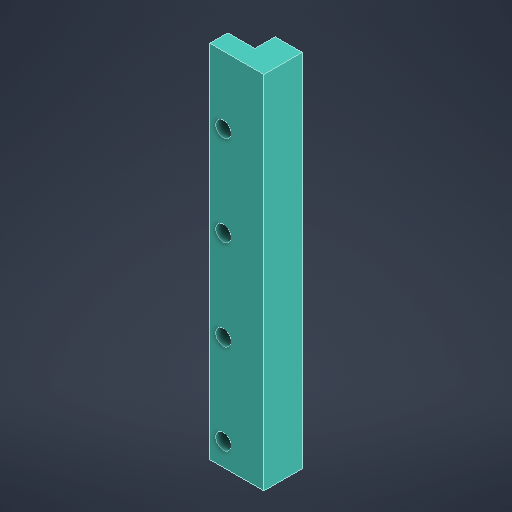
# Autodesk Inventor part: Left_Rod_Support
Saved by Autodesk Inventor 2027.1 (Build 311270010, 270A)
## iProperties
Created: 2026-09-22
Part Number: Left_Rod_Support
Material: Generic
Document SubType Name: Modeling
Designer: 박정현
Density: 1 g/cm^3
Appearance: Left separate support; four original rod clearance holes and four blind M3 x 0.5 - 6H deck threads, 6.5 mm depth.
Author: 박정현
Comments: Left separate support; four original rod clearance holes and four blind M3 x 0.5 - 6H deck threads, 6.5 mm depth.
Autodesk Inventor part; units mm, degrees
ref_plane "Left_Connecting_Web_StartPlane" through (0, 0, 4) normal (0, 0, 1) x (1, 0, 0)
sketch "Left_Connecting_Web_Profile" plane through (0, 0, 4) normal (0, 0, 1) x (1, 0, 0)
  line L0 (6, 0) -> (12, 0)
  line L1 (12, 0) -> (12, 80)
  line L2 (12, 80) -> (6, 80)
  line L3 (6, 80) -> (6, 0)
  point P0 (0, 0)
  dimension "d1" = 6
  dimension "d2" = 6
  dimension "d3" = 80
  constraints: 8 end point, 2 parallel, 1 horizontal, 1 horizontal alignment, 1 perpendicular
  measures "d1" distance of point (0, 0) L0.start
  measures "d2" distance of L1.end L2.end
  measures "d3" distance of L2.end L0.start
extrude "Left_Connecting_Web" add sketch "Left_Connecting_Web_Profile" along normal blind 8.5
ref_plane "Left_Rod_Contact_Flange_StartPlane" through (0, 0, 8.5) normal (0, 0, 1) x (1, 0, 0)
sketch "Left_Rod_Contact_Flange_Profile" plane through (0, 0, 8.5) normal (0, 0, 1) x (1, 0, 0)
  line L0 (0, 0) -> (12, 0)
  line L1 (12, 0) -> (12, 80)
  line L2 (12, 80) -> (0, 80)
  line L3 (0, 80) -> (0, 0)
  dimension "d7" = 12
  dimension "d8" = 80
  constraints: 8 end point, 2 parallel, 1 coincident, 1 horizontal, 1 perpendicular
  measures "d7" distance of L1.end L2.end
  measures "d8" distance of L2.end L0.start
extrude "Left_Rod_Contact_Flange" add sketch "Left_Rod_Contact_Flange_Profile" along normal blind 4
sketch "Original_Rod_Clearance_4x_Locations" plane through (0, 0, 0) normal (0, 0, 1) x (1, 0, 0)
  circle A0 centre (3, 5) radius 1.7
  circle A1 centre (3, 25) radius 1.7
  circle A2 centre (3, 45) radius 1.7
  circle A3 centre (3, 65) radius 1.7
  point P0 (0, 0)
  dimension "d11" = 3
  dimension "d12" = 5
  dimension "d13" = 3.4
  dimension "d14" = 3
  dimension "d15" = 25
  dimension "d16" = 3.4
  dimension "d17" = 3
  dimension "d18" = 45
  dimension "d19" = 3.4
  dimension "d20" = 3
  dimension "d21" = 65
  dimension "d22" = 3.4
  constraints: 4 centre point
  measures "d11" horizontal distance of point (0, 0) A0.centre
  measures "d12" vertical distance of point (0, 0) A0.centre
  measures "d13" diameter of A0
  measures "d14" horizontal distance of point (0, 0) A1.centre
  measures "d15" vertical distance of point (0, 0) A1.centre
  measures "d16" diameter of A1
  measures "d17" horizontal distance of point (0, 0) A2.centre
  measures "d18" vertical distance of point (0, 0) A2.centre
  measures "d19" diameter of A2
  measures "d20" horizontal distance of point (0, 0) A3.centre
  measures "d21" vertical distance of point (0, 0) A3.centre
  measures "d22" diameter of A3
extrude "Original_Rod_Clearance_4x" cut sketch "Original_Rod_Clearance_4x_Locations" along normal through all
ref_plane "Work Plane3" through (0, 0, 4) normal (0, 0, 1) x (1, 0, 0)
sketch "Deck_Assembly_M3_Locations" plane through (0, 0, 4) normal (0, 0, 1) x (1, 0, 0)
  circle A0 centre (9.5, 10) radius 1.25
  circle A1 centre (9.5, 30) radius 1.25
  circle A2 centre (9.5, 50) radius 1.25
  circle A3 centre (9.5, 70) radius 1.25
  point P0 (0, 0)
  dimension "d26" = 9.5
  dimension "d27" = 10
  dimension "d28" = 2.5
  dimension "d29" = 9.5
  dimension "d30" = 30
  dimension "d31" = 2.5
  dimension "d32" = 9.5
  dimension "d33" = 50
  dimension "d34" = 2.5
  dimension "d35" = 9.5
  dimension "d36" = 70
  dimension "d37" = 2.5
  constraints: 4 centre point
  measures "d26" horizontal distance of point (0, 0) A0.centre
  measures "d27" vertical distance of point (0, 0) A0.centre
  measures "d28" diameter of A0
  measures "d29" horizontal distance of point (0, 0) A1.centre
  measures "d30" vertical distance of point (0, 0) A1.centre
  measures "d31" diameter of A1
  measures "d32" horizontal distance of point (0, 0) A2.centre
  measures "d33" vertical distance of point (0, 0) A2.centre
  measures "d34" diameter of A2
  measures "d35" horizontal distance of point (0, 0) A3.centre
  measures "d36" vertical distance of point (0, 0) A3.centre
  measures "d37" diameter of A3
extrude "Four_Blind_M3_Tap_Bores" cut sketch "Deck_Assembly_M3_Locations" along normal blind 6.5
thread "Deck_M3x0_5_6H_1" size "M3x0.5" class "6H" standard "ISO Metric profile" length 6.5
thread "Deck_M3x0_5_6H_2" size "M3x0.5" class "6H" standard "ISO Metric profile" length 6.5
thread "Deck_M3x0_5_6H_3" size "M3x0.5" class "6H" standard "ISO Metric profile" length 6.5
thread "Deck_M3x0_5_6H_4" size "M3x0.5" class "6H" standard "ISO Metric profile" length 6.5
equation "\"d1\" = RodWidth"
equation "\"d2\" = WebThickness"
equation "\"d3\" = ContactLength"
equation "\"d4\" = DropHeight"
equation "\"d7\" = RodWidth + WebThickness"
equation "\"d8\" = ContactLength"
equation "\"d9\" = BaseThickness"
equation "\"d11\" = 0.5 * RodWidth"
equation "\"d12\" = RodHoleStart + 0 * RodScrewPitch"
equation "\"d13\" = RodClearanceDiameter"
equation "\"d14\" = 0.5 * RodWidth"
equation "\"d15\" = RodHoleStart + RodScrewPitch"
equation "\"d16\" = RodClearanceDiameter"
equation "\"d17\" = 0.5 * RodWidth"
equation "\"d18\" = RodHoleStart + 2 * RodScrewPitch"
equation "\"d19\" = RodClearanceDiameter"
equation "\"d20\" = 0.5 * RodWidth"
equation "\"d21\" = RodHoleStart + 3 * RodScrewPitch"
equation "\"d22\" = RodClearanceDiameter"
equation "\"d26\" = JoinLeftX"
equation "\"d27\" = JoinFirstY + 0 * JoinPitch"
equation "\"d28\" = TapDrillDiameter"
equation "\"d29\" = JoinLeftX"
equation "\"d30\" = JoinFirstY + JoinPitch"
equation "\"d31\" = TapDrillDiameter"
equation "\"d32\" = JoinLeftX"
equation "\"d33\" = JoinFirstY + 2 * JoinPitch"
equation "\"d34\" = TapDrillDiameter"
equation "\"d35\" = JoinLeftX"
equation "\"d36\" = JoinFirstY + 3 * JoinPitch"
equation "\"d37\" = TapDrillDiameter"
equation "\"d38\" = JoinThreadDepth"
equation "\"d40\" = JoinThreadDepth"
equation "\"d42\" = JoinThreadDepth"
equation "\"d44\" = JoinThreadDepth"
equation "\"d46\" = JoinThreadDepth"
equation "\"OverallWidth\" = 51"
equation "\"RodWidth\" = 6"
equation "\"ContactLength\" = 80"
equation "\"BaseThickness\" = 4"
equation "\"DropHeight\" = 8.5"
equation "\"WebThickness\" = 6"
equation "\"FingerStartX\" = 19.93338"
equation "\"FingerWidth\" = 13.5"
equation "\"FingerThickness\" = 6"
equation "\"FingerEndInset\" = 4"
equation "\"RodClearanceDiameter\" = 3.4"
equation "\"ClampFirstY\" = 41.82802"
equation "\"ClampPitch\" = 16"
equation "\"ClampHeight\" = BaseThickness + 0.5 * FingerThickness"
equation "\"TapDrillDiameter\" = 2.5"
equation "\"TapDepth\" = 6"
equation "\"RodHoleStart\" = 5"
equation "\"RodScrewPitch\" = 20"
equation "\"JoinLeftX\" = 9.5"
equation "\"JoinFirstY\" = 10"
equation "\"JoinPitch\" = 20"
equation "\"JoinThreadDepth\" = 6.5"
equation "\"JoinCountersinkDiameter\" = 6.2"
equation "\"d0\" = BaseThickness"
equation "\"d6\" = DropHeight"
equation "\"d25\" = BaseThickness"
body "Solid1"
